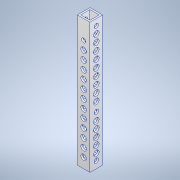
# Autodesk Inventor part: ハンド9x9_1_CPY
Saved by Autodesk Inventor 2020.3 (Build 243373000, 373)
## iProperties
Created: 2020-05-31
Part Number: ハンド9x9_1_CPY
Material: アルミニウム 6061
Document SubType Name: Modeling
Designer: totot
Mass: 6.90377 g
Surface Area: 52.5331 cm^2
Volume: 2.55695 cm^3
Density: 2.7 g/cm^3
Appearance: アルミニウム - フラット
Author: totot
Autodesk Inventor part; units mm, degrees
ref_plane "YZ Plane" through (0, 0, 0) normal (1, 0, 0) x (0, 1, 0)
ref_plane "XZ Plane" through (0, 0, 0) normal (0, 1, 0) x (-1, 0, 0)
ref_plane "XY Plane" through (0, 0, 0) normal (0, 0, 1) x (1, 0, 0)
sketch "スケッチ1" plane through (0, 0, 0) normal (0, 1, 0) x (-1, 0, 0)
  line L0 (0, 0) -> (-9, 0)
  line L1 (-9, 0) -> (-9, 9)
  line L2 (-9, 9) -> (0, 9)
  line L3 (0, 9) -> (0, 0)
  line L4 (-1.2, 7.8) -> (-7.8, 7.8)
  line L5 (-7.8, 7.8) -> (-7.8, 1.2)
  line L6 (-7.8, 1.2) -> (-1.2, 1.2)
  line L7 (-1.2, 1.2) -> (-1.2, 7.8)
  dimension "d0" = 9
  dimension "d1" = 9
  dimension "d2" = 1.2
  dimension "d3" = 1.2
  dimension "d4" = 1.2
  dimension "d5" = 1.2
  constraints: 16 end point, 4 parallel, 2 horizontal, 2 perpendicular
  measures "d0" distance of L1.end L2.end
  measures "d1" distance of L0.end L1.end
  measures "d2" distance between parallel lines of L3 L7
  measures "d3" distance between parallel lines of L2 L4
  measures "d4" distance between parallel lines of L6 L0
  measures "d5" distance between parallel lines of L1 L5
extrude "押し出し1" add sketch "スケッチ1" along normal blind 92.5
sketch "スケッチ2" plane through (9, 0, 9) normal (1, 0, 0) x (0, 0, -1)
  line L0 (0, 0) -> (9, 0) projected
  line L1 (0, 0) -> (0, 92.5) projected
  point P0 (4.5, 5)
  point P1 (4.5, 35)
  dimension "d8" = 30
  dimension "d9" = 5
  dimension "d10" = 4.5
  dimension "d11" = 4.5
  measures "d8" distance of point (4.5, 5) point (4.5, 35)
  measures "d9" distance from line of L0 point (4.5, 5)
  measures "d10" distance from line of L1 point (4.5, 35)
  measures "d11" distance from line of L1 point (4.5, 5)
hole "穴1" at (9, 5, 4.5) at (9, 35, 4.5) direction (-1, 0, 0) diameter 3.3 end through all
sketch "スケッチ5" plane through (9, 0, 0) normal (0, 0, -1) x (-1, 0, 0)
  line L0 (0, 92.5) -> (9, 92.5) projected
  line L1 (9, 0) -> (9, 92.5) projected
  point P0 (4.5, 79)
  dimension "d41" = 13.5
  dimension "d42" = 4.5
  measures "d41" distance from line of point (4.5, 79) L0
  measures "d42" distance from line of point (4.5, 79) L1
hole "穴4" at (4.5, 79, 0) direction (0, 0, 1) diameter 3 end through all
sketch "スケッチ6" plane through (0, 0, 0) normal (-1, 0, 0) x (0, 0, 1)
  line L0 (0, 92.5) -> (9, 92.5) projected
  line L1 (0, 0) -> (0, 92.5) projected
  point P0 (4.5, 88)
  dimension "d50" = 4.5
  dimension "d51" = 4.5
  measures "d50" distance from line of point (4.5, 88) L0
  measures "d51" distance from line of L1 point (4.5, 88)
hole "穴5" at (0, 88, 4.5) direction (1, 0, 0) diameter 3 end through all
sketch "スケッチ7" plane through (0, 0, 9) normal (0, 0, 1) x (1, 0, 0)
  circle A0 centre (4.5, 79) radius 1.5 projected
  line L0 (0, 0) -> (0, 92.5) projected
  point P0 (4.5, 73)
  point P1 (4.5, 67)
  point P2 (4.5, 61)
  point P3 (4.5, 55)
  point P4 (4.5, 49)
  point P5 (4.5, 43)
  point P6 (4.5, 37)
  point P7 (4.5, 31)
  point P8 (4.5, 25)
  point P9 (4.5, 19)
  point P10 (4.5, 13)
  point P11 (4.5, 7)
  dimension "d59" = 6
  dimension "d60" = 4.5
  dimension "d63" = 6
  dimension "d70" = 6
  dimension "d77" = 6
  constraints: 3 vertical, 11 other
  measures "d59" distance of point (4.5, 73) A0.centre
  measures "d60" distance from line of point (4.5, 73) L0
  measures "d63" distance of point (4.5, 73) point (4.5, 67)
  measures "d70" distance of point (4.5, 49) point (4.5, 43)
  measures "d77" distance of point (4.5, 25) point (4.5, 19)
hole "穴6" at (4.5, 73, 9) at (4.5, 67, 9) at (4.5, 61, 9) at (4.5, 55, 9) at (4.5, 49, 9) at (4.5, 43, 9) at (4.5, 37, 9) at (4.5, 31, 9) at (4.5, 25, 9) at (4.5, 19, 9) at (4.5, 13, 9) at (4.5, 7, 9) direction (0, 0, -1) diameter 4 end through all
sketch "スケッチ8" plane through (9, 0, 9) normal (1, 0, 0) x (0, 0, -1)
  line L0 (0, 0) -> (0, 92.5) projected
  circle A0 centre (4.5, 5) radius 1.65 projected
  point P0 (9, 0)
  point P1 (4.5, 9.5)
  point P2 (4.5, 14.5)
  point P3 (4.5, 19.5)
  point P4 (4.5, 24.5)
  point P5 (4.5, 29.5)
  dimension "d89" = 4.5
  dimension "d90" = 4.5
  dimension "d93" = 5
  constraints: 1 vertical, 4 other
  measures "d89" distance from line of point (4.5, 9.5) L0
  measures "d90" distance of point (4.5, 9.5) A0.centre
  measures "d93" distance of point (4.5, 9.5) point (4.5, 14.5)
hole "穴7" at (9, 9.5, 4.5) at (9, 14.5, 4.5) at (9, 19.5, 4.5) at (9, 24.5, 4.5) at (9, 29.5, 4.5) direction (-1, 0, 0) diameter 4 end through all
sketch "スケッチ9" plane through (9, 0, 9) normal (1, 0, 0) x (0, 0, -1)
  line L0 (0, 0) -> (0, 92.5) projected
  circle A0 centre (4.5, 88) radius 1.5 projected
  point P0 (9, 0)
  point P1 (4.5, 83)
  point P2 (4.5, 77.8)
  point P3 (4.5, 72.6)
  point P4 (4.5, 67.4)
  point P5 (4.5, 62.2)
  point P6 (4.5, 57)
  point P7 (4.5, 51.8)
  point P8 (4.5, 46.6)
  point P9 (4.5, 41.4)
  dimension "d105" = 4.5
  dimension "d106" = 5
  dimension "d109" = 5.2
  constraints: 1 vertical, 8 other
  measures "d105" distance from line of point (4.5, 83) L0
  measures "d106" distance of point (4.5, 83) A0.centre
  measures "d109" distance of point (4.5, 83) point (4.5, 77.8)
hole "穴8" at (9, 83, 4.5) at (9, 77.8, 4.5) at (9, 72.6, 4.5) at (9, 67.4, 4.5) at (9, 62.2, 4.5) at (9, 57, 4.5) at (9, 51.8, 4.5) at (9, 46.6, 4.5) at (9, 41.4, 4.5) direction (-1, 0, 0) diameter 4 end through all
sketch "スケッチ10" plane through (0, 0, 9) normal (0, 0, 1) x (1, 0, 0)
  line L0 (9, 0) -> (9, 92.5) projected
  line L1 (0, 92.5) -> (9, 92.5) projected
  point P0 (0, 0)
  point P1 (4.5, 85.75)
  dimension "d121" = 4.5
  dimension "d122" = 6.75
  measures "d121" distance from line of point (4.5, 85.75) L0
  measures "d122" distance from line of point (4.5, 85.75) L1
hole "穴9" at (4.5, 85.75, 9) direction (0, 0, -1) diameter 5 end through all
equation "\"d3\" = d2"
equation "\"d4\" = d2"
equation "\"d5\" = d3"
equation "\"d51\" = d50"
